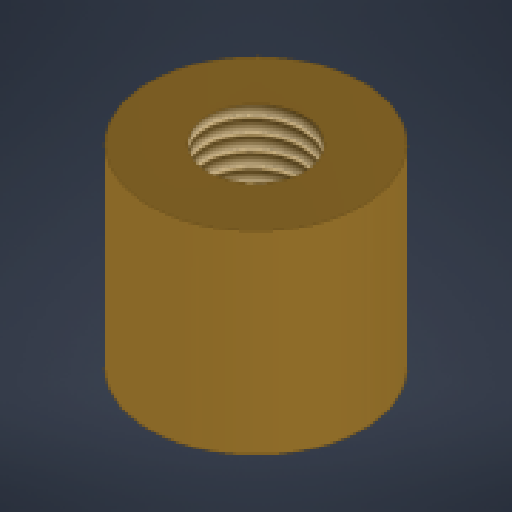
# Autodesk Inventor part: SpindleBlock_V1
Saved by Autodesk Inventor 2024.1 (Build 281209000, 209)
## iProperties
Created: 2022-11-22
Part Number: SpindleBlock_V1
Material: Brass, Soft Yellow
Document SubType Name: Modeling
Designer: jaege
Density: 8.47 g/cm^3
Appearance: Brass - Satin
Author: jaege
Autodesk Inventor part; units mm, degrees
ref_plane "YZ Plane" through (0, 0, 0) normal (1, 0, 0) x (0, 1, 0)
ref_plane "XZ Plane" through (0, 0, 0) normal (0, 1, 0) x (-1, 0, 0)
ref_plane "XY Plane" through (0, 0, 0) normal (0, 0, 1) x (1, 0, 0)
sketch "Sketch1" plane through (0, 0, 0) normal (0, 1, 0) x (-1, 0, 0)
  circle A0 centre (0, 0) radius 5
  circle A1 centre (0, 0) radius 11
  dimension "d0" = 10
  dimension "d1" = 22
  constraints: 2 centre point, 2 coincident
  measures "d0" diameter of A0
  measures "d1" diameter of A1
extrude "Extrusion1" add sketch "Sketch1" along normal blind 20
thread "Thread1" size "M10x1.5" class "6H" standard "ANSI Metric M Profile" full length
body "Solid1"
